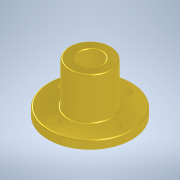
# Autodesk Inventor part: Trapezmutter_T8
Saved by Autodesk Inventor 2021 (Build 250183000, 183)
## iProperties
Created: 2021-04-21
Part Number: Trapezmutter_T8
Material: Generic
Document SubType Name: Modeling
Designer: Fabijan_Sven
Density: 1 g/cm^3
Appearance: Metal 2400F Hot
Author: Fabijan_Sven
Autodesk Inventor part; units mm, degrees
ref_plane "YZ Plane" through (0, 0, 0) normal (1, 0, 0) x (0, 1, 0)
ref_plane "XZ Plane" through (0, 0, 0) normal (0, 1, 0) x (-1, 0, 0)
ref_plane "XY Plane" through (0, 0, 0) normal (0, 0, 1) x (1, 0, 0)
sketch "Sketch1" plane through (0, 0, 0) normal (0, 1, 0) x (-1, 0, 0)
  circle A0 centre (0, 0) radius 15
  dimension "d0" = 30
  constraints: 1 centre point, 1 coincident
  measures "d0" diameter of A0
extrude "Extrusion1" add sketch "Sketch1" along normal blind 5
sketch "Sketch2" plane through (0, 5, 0) normal (0, 1, 0) x (1, 0, 0)
  circle A0 centre (0, 0) radius 6.5
  dimension "d3" = 13
  constraints: 1 centre point, 1 coincident
  measures "d3" diameter of A0
extrude "Extrusion2" add sketch "Sketch2" along normal blind 15
sketch "Sketch3" plane through (0, 20, 0) normal (0, 1, 0) x (1, 0, 0)
  point P0 (0, 0)
hole "Hole1" at (0, 20, 0) direction (0, -1, 0) diameter 8 end through all
fillet "Fillet1" radius 0.5 6 edges at (-6.5, 20, 0) (0, 20, -4) (-6.5, 5, 0) (15, 5, 0) (15, 0, 0) (0, 0, -4)
sketch "Sketch4" plane through (0, 5, 0) normal (0, 1, 0) x (1, 0, 0)
  circle A0 centre (0, 0) radius 11
  circle A1 centre (-1.7851, -10.8542) radius 2
  circle A2 centre (10.8542, -1.7851) radius 2
  circle A3 centre (1.7851, 10.8542) radius 2
  circle A4 centre (-10.8542, 1.7851) radius 2
  dimension "d14" = 22
  dimension "d15" = 4
  dimension "d18" = 360
  constraints: 4 centre point, 3 coincident, 14 other
  measures "d15" diameter of A1
hole "Hole2" at (-1.7851, 5, 10.8542) at (10.8542, 5, 1.7851) at (1.7851, 5, -10.8542) at (-10.8542, 5, -1.7851) direction (0, -1, 0) diameter 4 end through all
sketch "Sketch5" plane through (0, 0, 0) normal (0, -1, 0) x (1, 0, 0)
  circle A0 centre (0, 0) radius 6
  circle A1 centre (0, 0) radius 16
  dimension "d27" = 12
  dimension "d28" = 32
  constraints: 2 centre point, 2 coincident
  measures "d27" diameter of A0
  measures "d28" diameter of A1
extrude "Extrusion3" cut sketch "Sketch5" against normal blind 2
sketch "Sketch6" plane through (0, 2, 0) normal (0, -1, 0) x (1, 0, 0)
  circle A0 centre (0, 0) radius 8
  circle A1 centre (0, 0) radius 16.0389
  dimension "d31" = 16
  dimension "d32" = 32.0778
  constraints: 2 centre point, 2 coincident
  measures "d31" diameter of A0
  measures "d32" diameter of A1
extrude "Extrusion4" cut sketch "Sketch6" against normal up to surface (3 mm away)
fillet "Fillet2" radius 0.5 2 edges at (-8, 2, 0) (-6, 0, 0)
body "Solid1"
